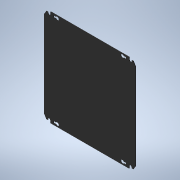
# Autodesk Inventor part: 155X_02_00_P6_(1)
Saved by Autodesk Inventor 2021 (Build 250183000, 183)
## iProperties
Created: 2025-07-29
Part Number: 155X_02_00_P6_(1)
Material: Generic
Catalog Web Link: www.cadenas.de
Description: AE 2.0 Montageplatte-AE 2.0 Montageplatte
Vendor: RITTAL
Document SubType Name: Modeling
Designer: psAdmin
Manufacturer: RITTAL
Mass: 527.052 g
Surface Area: 4270.76 cm^2
Volume: 527.052 cm^3
Density: 1 g/cm^3
Appearance: PSOLRGB-176-176-176
Category: PARTsolutions
Company: RITTAL
Title: 155X_02_00_P6
Author: Cadenas PARTsolutions
Comments: AE 2.0 Montageplatte
PSOL_IDENT_0: {$CADENAS_DATA/23d-libs/rittal/schaltschranksys/kompakt_schaltschr/parts_ae_2_0/montageplatte_ae_2_0
PSOL_IDENT_1: .prj},197 {VTYP=3D},{NB=155X_02_00_P6_(1)},{LINA=155X_02_00_P6},{NN=AE 2.0 Montageplatte},{DATE=28.0
PSOL_IDENT_2: 4.2025 21:11:32},{GEOMDATE=11.04.2025 07:46:14},{VERSION=},{LINEID=180},{WBVAR=DETAIL},{WBNUMERIC=DE
PSOL_IDENT_3: TAIL}  {NB=155X_02_00_P6_(1)},{LINA=155X_02_00_P6},{KT=DUMMY},{BEST=155X},{B=500},{H=500},{S=2.5},{T=
PSOL_IDENT_4: MIN},{B1=450},{H1=475},{VERS=3},{DETAIL=1},{BEZ1=Neues Kompaktgehäuse},{BEZ2=Stahlblech},{BEZ3=eintü
PSOL_IDENT_5: rig},{F=450},{G=475},{CNSECLASS51=27-18-01-02},{CNSECLASS70=27-18-01-01},{CNSECLASS80=27-18-01-01},{
PSOL_IDENT_6: CNSETIM40=EC000261}
NB: 155X_02_00_P6_(1)
NN: AE 2.0 Montageplatte
NT: AE 2.0 Montageplatte
NBSYN: $BEST._02_00_P6_($DETAIL.)
LINA: 155X_02_00_P6
CATALOG: Rittal
BEST: 155X
B: 500
H: 500
S: 2.5
T: 0
B1: 450
H1: 475
VERS: 3
DETAIL: hoch
BEZ1: Neues Kompaktgehäuse
BEZ2: Stahlblech
BEZ3: eintürig
F: 450
G: 475
CNSECLASS70: 27-18-01-01
CNSECLASS80: 27-18-01-01
SUPPLIER: RITTAL
ARTICLENO: 155X_02_00_P6_(1)
BOMINFO: 155X_02_00_P6
CREATOR: CADENAS GmbH
Autodesk Inventor part; units mm, degrees
sketch "Sketch_11" plane through (0, 0, 0) normal (0, 0, 1) x (1, 0, 0)
  line L0 (-225, 438.5) -> (-225, 11.5)
  line L1 (-225, 11.5) -> (-224.0774, 11.5)
  arc A0 (-223.2113, 11) -> (-224.0774, 11.5) centre (-224.0774, 10.5) ccw
  line L2 (-223.2113, 11) -> (-214.2624, -4.5)
  arc A1 (-214.2624, -4.5) -> (-213.3964, -5) centre (-213.3964, -4) ccw
  line L3 (-213.3964, -5) -> (-206.5, -5)
  arc A2 (-206.5, -5) -> (-205.5, -4) centre (-206.5, -4) ccw
  line L4 (-205.5, -4) -> (-205.5, 0)
  arc A3 (-194.5, 0) -> (-205.5, 0) centre (-200, 0) ccw
  line L5 (-194.5, 0) -> (-194.5, -11)
  line L6 (-194.5, -11) -> (-193, -12.5)
  line L7 (-193, -12.5) -> (193, -12.5)
  line L8 (193, -12.5) -> (194.5, -11)
  line L9 (194.5, -11) -> (194.5, 0)
  arc A4 (205.5, 0) -> (194.5, 0) centre (200, 0) ccw
  line L10 (205.5, 0) -> (205.5, -4)
  arc A5 (205.5, -4) -> (206.5, -5) centre (206.5, -4) ccw
  line L11 (206.5, -5) -> (213.3964, -5)
  arc A6 (213.3964, -5) -> (214.2624, -4.5) centre (213.3964, -4) ccw
  line L12 (214.2624, -4.5) -> (223.2113, 11)
  arc A7 (224.0774, 11.5) -> (223.2113, 11) centre (224.0774, 10.5) ccw
  line L13 (224.0774, 11.5) -> (225, 11.5)
  line L14 (225, 11.5) -> (225, 438.5)
  line L15 (225, 438.5) -> (224.0774, 438.5)
  arc A8 (223.2113, 439) -> (224.0774, 438.5) centre (224.0774, 439.5) ccw
  line L16 (223.2113, 439) -> (214.2624, 454.5)
  arc A9 (214.2624, 454.5) -> (213.3964, 455) centre (213.3964, 454) ccw
  line L17 (213.3964, 455) -> (206.5, 455)
  arc A10 (206.5, 455) -> (205.5, 454) centre (206.5, 454) ccw
  line L18 (205.5, 454) -> (205.5, 450)
  arc A11 (194.5, 450) -> (205.5, 450) centre (200, 450) ccw
  line L19 (194.5, 450) -> (194.5, 461)
  line L20 (194.5, 461) -> (193, 462.5)
  line L21 (193, 462.5) -> (-193, 462.5)
  line L22 (-193, 462.5) -> (-194.5, 461)
  line L23 (-194.5, 461) -> (-194.5, 450)
  arc A12 (-205.5, 450) -> (-194.5, 450) centre (-200, 450) ccw
  line L24 (-205.5, 450) -> (-205.5, 454)
  arc A13 (-205.5, 454) -> (-206.5, 455) centre (-206.5, 454) ccw
  line L25 (-206.5, 455) -> (-213.3964, 455)
  arc A14 (-213.3964, 455) -> (-214.2624, 454.5) centre (-213.3964, 454) ccw
  line L26 (-214.2624, 454.5) -> (-223.2113, 439)
  arc A15 (-224.0774, 438.5) -> (-223.2113, 439) centre (-224.0774, 439.5) ccw
  line L27 (-224.0774, 438.5) -> (-225, 438.5)
  arc A16 (166.5296, 4.6222) -> (166.5296, -4.6222) centre (160, 0) ccw
  arc A17 (167.3457, -4.2) -> (166.5296, -4.6222) centre (167.3457, -5.2) ccw
  line L28 (167.3457, -4.2) -> (178, -4.2)
  arc A18 (178, -4.2) -> (179, -3.2) centre (178, -3.2) ccw
  line L29 (179, -3.2) -> (179, 3.2)
  arc A19 (179, 3.2) -> (178, 4.2) centre (178, 3.2) ccw
  line L30 (178, 4.2) -> (167.3457, 4.2)
  arc A20 (166.5296, 4.6222) -> (167.3457, 4.2) centre (167.3457, 5.2) ccw
  arc A21 (166.5296, 454.6222) -> (166.5296, 445.3778) centre (160, 450) ccw
  arc A22 (167.3457, 445.8) -> (166.5296, 445.3778) centre (167.3457, 444.8) ccw
  line L31 (167.3457, 445.8) -> (178, 445.8)
  arc A23 (178, 445.8) -> (179, 446.8) centre (178, 446.8) ccw
  line L32 (179, 446.8) -> (179, 453.2)
  arc A24 (179, 453.2) -> (178, 454.2) centre (178, 453.2) ccw
  line L33 (178, 454.2) -> (167.3457, 454.2)
  arc A25 (166.5296, 454.6222) -> (167.3457, 454.2) centre (167.3457, 455.2) ccw
  line L34 (-179, 3.2) -> (-179, -3.2)
  arc A26 (-179, -3.2) -> (-178, -4.2) centre (-178, -3.2) ccw
  line L35 (-178, -4.2) -> (-167.3457, -4.2)
  arc A27 (-166.5296, -4.6222) -> (-167.3457, -4.2) centre (-167.3457, -5.2) ccw
  arc A28 (-166.5296, -4.6222) -> (-166.5296, 4.6222) centre (-160, 0) ccw
  arc A29 (-167.3457, 4.2) -> (-166.5296, 4.6222) centre (-167.3457, 5.2) ccw
  line L36 (-167.3457, 4.2) -> (-178, 4.2)
  arc A30 (-178, 4.2) -> (-179, 3.2) centre (-178, 3.2) ccw
  arc A31 (-179, 446.8) -> (-178, 445.8) centre (-178, 446.8) ccw
  line L37 (-178, 445.8) -> (-167.3457, 445.8)
  arc A32 (-166.5296, 445.3778) -> (-167.3457, 445.8) centre (-167.3457, 444.8) ccw
  arc A33 (-166.5296, 445.3778) -> (-166.5296, 454.6222) centre (-160, 450) ccw
  arc A34 (-167.3457, 454.2) -> (-166.5296, 454.6222) centre (-167.3457, 455.2) ccw
  line L38 (-167.3457, 454.2) -> (-178, 454.2)
  arc A35 (-178, 454.2) -> (-179, 453.2) centre (-178, 453.2) ccw
  line L39 (-179, 453.2) -> (-179, 446.8)
  constraints: 80 end point, 72 point on circle, 36 centre point
extrude "Extrusion1" add sketch "Sketch_11" against normal blind 2.5
ref_plane "MP_XY" through (0, 0, 0) normal (0, 0, 1) x (1, 0, 0)
ref_plane "MP_YZ" through (0, 0, 0) normal (1, 0, 0) x (0, 1, 0)
ref_plane "MP_ZX" through (0, 0, 0) normal (0, 1, 0) x (0, 0, 1)
ref_plane "to_EB_XY" through (174.8, 0, -2.5) normal (0, 0, 1) x (1, 0, 0)
ref_plane "to_EB_YZ" through (174.8, 0, -2.5) normal (1, 0, 0) x (0, 1, 0)
ref_plane "to_EB_ZX" through (174.8, 0, -2.5) normal (0, 1, 0) x (0, 0, 1)
body "Solid1"
